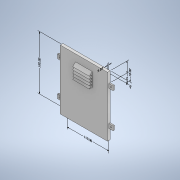
# Autodesk Inventor part: caseDoor
Saved by Autodesk Inventor 2022.6 (Build 266554010, 554A)
## iProperties
Created: 2025-03-20
Part Number: caseDoor
Material: Generic
Document SubType Name: Modeling
Designer: khinm
Density: 1 g/cm^3
Appearance: Default
Author: khinm
Autodesk Inventor part; units mm, degrees
sketch "Sketch1" plane through (0, 0, 0) normal (1, 0, 0) x (0, 1, 0)
  line L0 (215, 0) -> (0, 0)
  line L1 (0, 0) -> (0, -15)
  line L2 (0, -15) -> (215, -15)
  line L3 (215, -15) -> (215, 0)
  dimension "d0" = 15
  dimension "d1" = 215
  constraints: 8 end point, 2 parallel, 1 coincident, 1 horizontal, 1 perpendicular
  measures "d0" distance of L2.end L0.start
  measures "d1" distance of L1.end L2.end
extrude "Extrusion1" add sketch "Sketch1" along normal mid plane 170
sketch "Sketch2" plane through (85, 0, 0) normal (1, 0, 0) x (0, 0, -1)
  line L0 (15, 0) -> (15, 215) projected
  line L1 (15, 215) -> (0, 215) projected
  line L2 (15, 215) -> (10, 215)
  line L3 (10, 215) -> (10, 205)
  line L4 (10, 205) -> (15, 205)
  line L5 (15, 205) -> (15, 215)
  point P0 (0, 0)
  point P1 (12.5, 215)
  point P2 (12.5, 205)
  point P3 (15, 210)
  point P4 (10, 210)
  point P5 (15, 205)
  dimension "d4" = 10
  dimension "d5" = 5
  constraints: 8 end point, 4 midpoint, 2 parallel, 1 horizontal, 1 perpendicular
  measures "d4" distance of point (12.5, 215) point (12.5, 205)
  measures "d5" distance of point (15, 210) point (10, 210)
sketch3d "3D Sketch1"
  line L0 (85, 215, -15) -> (-85, 215, -15)
  line L1 (-85, 215, -15) -> (-85, 0, -15)
  line L2 (-85, 0, -15) -> (85, 0, -15)
  line L3 (85, 0, -15) -> (85, 215, -15)
sweep "Sweep1" cut profiles "Sketch2" path "3D Sketch1"
ref_plane "Work Plane1" through (0, 0, 0) normal (1, 0, 0) x (0, 1, 0)
sketch "Sketch3" plane through (0, 0, 0) normal (1, 0, 0) x (0, 1, 0)
  line L0 (0, 0) -> (215, 0) projected
  line L1 (190, 0) -> (180, 0)
  line L2 (180, 0) -> (180, 10)
  line L3 (180, 10) -> (190, 0)
  point P0 (180, 5)
  dimension "d9" = 25
  dimension "d10" = 10
  dimension "d11" = 10
  constraints: 6 end point, 2 point on line, 1 midpoint, 1 vertical
  measures "d9" distance of L0.end L1.start
  measures "d10" horizontal distance of L1.start point (180, 5)
  measures "d11" distance of L1.end L2.end
extrude "Extrusion2" add sketch "Sketch3" along normal mid plane 60
sketch "Sketch4" plane through (0, 0, 0) normal (1, 0, 0) x (0, 1, 0)
  line L0 (10, -15) -> (205, -15) projected
  line L1 (180, -15) -> (180, 5)
  line L2 (180, 5) -> (185, 0)
  line L3 (185, 0) -> (185, -15)
  line L4 (185, -15) -> (180, -15)
  line L5 (180, 10) -> (190, 0) projected
  point P0 (0, 0)
  dimension "d14" = 5
  dimension "d15" = 5
  constraints: 8 end point, 2 point on line, 1 collinear, 1 parallel, 1 perpendicular, 1 vertical, 1 vertical alignment
  measures "d14" distance of L3.end L1.start
  measures "d15" distance of L5.start L1.end
extrude "Extrusion3" cut sketch "Sketch4" along normal mid plane 50
pattern_linear "Rectangular Pattern1" count 5 spacing 10 along (0, -1, 0) of "Extrusion2", "Extrusion3"
sketch "Sketch5" plane through (85, 0, 0) normal (1, 0, 0) x (0, 0, -1)
  line L0 (10, 0) -> (10, 215) projected
  line L1 (10, 10) -> (10, 205) projected
  line L2 (10, 177.5) -> (5, 177.5)
  line L3 (5, 177.5) -> (5, 162.5)
  line L4 (5, 162.5) -> (10, 162.5)
  line L5 (10, 162.5) -> (10, 177.5)
  point P0 (0, 0)
  point P1 (7.5, 177.5)
  point P2 (10, 177.5)
  point P3 (7.5, 162.5)
  dimension "d22" = 5
  dimension "d23" = 15
  dimension "d39" = 52.5
  constraints: 8 end point, 2 midpoint, 2 parallel, 1 horizontal, 1 perpendicular, 1 point on line
  measures "d22" distance of L4.end L3.end
  measures "d23" distance of L2.start L4.end
  measures "d39" vertical distance of L0.end point (7.5, 162.5)
extrude "Extrusion4" add sketch "Sketch5" along normal blind 15
sketch "Sketch6" plane through (85, 162.5, -5) normal (0, 0, 1) x (1, 0, 0)
  line L0 (0, 15) -> (15, 15) projected
  line L1 (15, 15) -> (15, 0) projected
  point P0 (-85, -162.5)
  point P1 (7.5, 7.5)
  point P2 (7.5, 15)
  point P3 (15, 7.5)
  dimension "d26" = 7.5
  dimension "d27" = 7.5
  constraints: 2 midpoint
  measures "d26" distance of point (7.5, 15) point (7.5, 7.5)
  measures "d27" distance of point (15, 7.5) point (7.5, 7.5)
hole "Hole1" at (92.5, 170, -5) direction (0, 0, -1) diameter 4.134 depth 5
ref_plane "Work Plane2" through (0, 107.5, 0) normal (0, 1, 0) x (-1, 0, 0)
mirror "Mirror1" about plane through (0, 107.5, 0) normal (0, 1, 0) of "Extrusion4", "Hole1"
ref_plane "Work Plane3" through (0, 0, 0) normal (0, 1, 0) x (-1, 0, 0)
ref_plane "Work Plane5" through (0, 0, 0) normal (1, 0, 0) x (0, 1, 0)
mirror "Mirror2" about plane through (0, 0, 0) normal (1, 0, 0) of "Extrusion4", "Hole1", "Mirror1"
body "Solid1"
